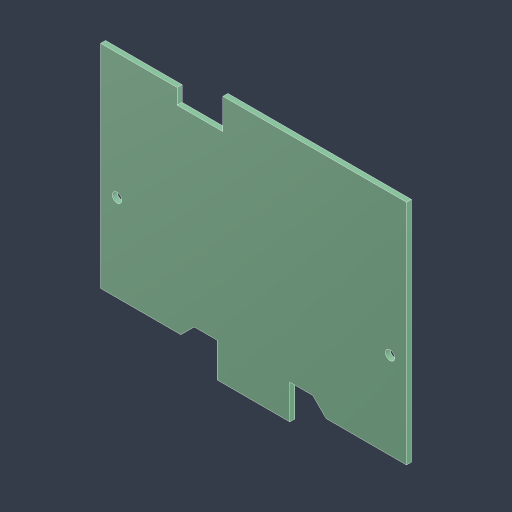
# Autodesk Inventor part: BDM-030
Saved by Autodesk Inventor 2023.4 (Build 274418000, 418)
## iProperties
Created: 2024-02-22
Part Number: BDM-030
Material: Generic
Document SubType Name: Modeling
Designer: JoaoSilva
Density: 1 g/cm^3
Appearance: Smooth - Dark Sea Green
Author: JoaoSilva
Autodesk Inventor part; units mm, degrees
ref_plane "YZ Plane" through (0, 0, 0) normal (1, 0, 0) x (0, 1, 0)
ref_plane "XZ Plane" through (0, 0, 0) normal (0, 1, 0) x (-1, 0, 0)
ref_plane "XY Plane" through (0, 0, 0) normal (0, 0, 1) x (1, 0, 0)
sketch "Sketch1" plane through (0, 0, 0) normal (0, 0, 1) x (1, 0, 0)
  line L0 (-40, 32.5) -> (40, 32.5)
  line L1 (40, 32.5) -> (40, -32.5)
  line L2 (40, -32.5) -> (-40, -32.5)
  line L3 (-40, -32.5) -> (-40, 32.5)
  line L4 (-40, 32.5) -> (40, -32.5) construction
  line L5 (40, 32.5) -> (-40, -32.5) construction
  line L6 (-8, 32.5) -> (-8, 24.5)
  line L7 (-8, 24.5) -> (-20, 24.5)
  line L8 (-20, 24.5) -> (-20, 28.5)
  line L9 (-20, 28.5) -> (-40, 28.5)
  line L10 (-40, -27) -> (-19, -27)
  line L11 (-19, -27) -> (-15.5, -23.5)
  line L12 (-15.5, -23.5) -> (-9.5, -23.5)
  line L13 (-9.5, -23.5) -> (-9.5, -32.5)
  line L14 (9.5, -32.5) -> (9.5, -23.5)
  line L15 (9.5, -23.5) -> (15.5, -23.5)
  line L16 (15.5, -23.5) -> (19, -27)
  line L17 (19, -27) -> (40, -27)
  point P0 (0, 0)
  dimension "d0" = 80
  dimension "d1" = 65
  dimension "d2" = 19
  dimension "d3" = 45
  dimension "d4" = 9
  dimension "d5" = 3.5
  dimension "d6" = 6
  dimension "d7" = 45
  dimension "d8" = 8
  dimension "d9" = 8
  dimension "d10" = 12
  dimension "d11" = 4
  constraints: 36 end point, 9 perpendicular, 6 point on line, 4 equal length, 3 parallel, 2 midpoint, 1 horizontal, 1 vertical
  measures "d0" distance of L1.end L2.end
  measures "d1" distance of L0.end L1.end
  measures "d2" distance between parallel lines of L14 L13
  measures "d3" angle of L10 L11
  measures "d4" distance of L12.end L13.end
  measures "d5" distance between parallel lines of L12 L10
  measures "d6" distance of L11.end L12.end
  measures "d7" angle of L17 L16
  measures "d8" distance from line of point (0, 0) L6
  measures "d9" distance of L6.start L6.end
  measures "d10" distance of L6.end L7.end
  measures "d11" distance between parallel lines of L7 L9
extrude "Extrusion1" add sketch "Sketch1" along normal blind 1.3 contours L0 L1 L17 L16 L15 L14 L2 L13 L12 L11 L10 L3 L9 L8 L7 L6
sketch "Sketch2" plane through (0, 0, 1.3) normal (0, 0, 1) x (1, 0, 0)
  line L0 (-35.7, -4.3) -> (35.7, -4.3) construction
  line L1 (-40, -27) -> (-19, -27) projected
  point P0 (0, 0)
  point P1 (0, -4.3)
  dimension "d14" = 71.4
  dimension "d15" = 22.7
  constraints: 2 end point, 1 horizontal, 1 midpoint, 1 vertical alignment
  measures "d14" distance of L0.start L0.end
  measures "d15" distance between parallel lines of L1 L0
hole "Hole1" at (-35.7, -4.3, 1.3) at (35.7, -4.3, 1.3) direction (0, 0, -1) diameter 2.5 end through all
equation "\"d7\" = d3"
body "Solid1"
